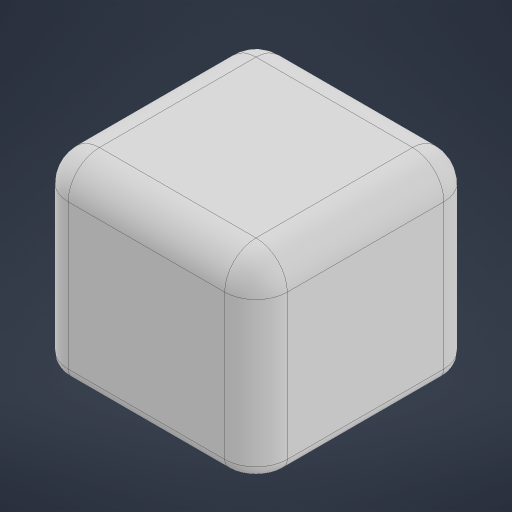
# Autodesk Inventor part: Cap
Saved by Autodesk Inventor 2024.1 (Build 281209000, 209)
## iProperties
Created: 2024-04-25
Part Number: Cap
Material: Generic
Document SubType Name: Modeling
Designer: Tim Jäger
Density: 1 g/cm^3
Appearance: Default
Author: Tim Jäger
## iProperties of the stored document Cap_3DPrint.ipt
Created: 2024-04-25
Part Number: Cap_3DPrint
Material: Generic
Document SubType Name: Modeling
Designer: Tim Jäger
Density: 1 g/cm^3
Appearance: Default
Author: Tim Jäger
Autodesk Inventor part; units mm, degrees
ref_plane "YZ Plane" through (0, 0, 0) normal (1, 0, 0) x (0, 1, 0)
ref_plane "XZ Plane" through (0, 0, 0) normal (0, 1, 0) x (-1, 0, 0)
ref_plane "XY Plane" through (0, 0, 0) normal (0, 0, 1) x (1, 0, 0)
sketch "Sketch1" plane through (0, 0, 0) normal (0, 1, 0) x (-1, 0, 0)
  line L0 (-10, 10) -> (10, 10)
  line L1 (10, 10) -> (10, -10)
  line L2 (10, -10) -> (-10, -10)
  line L3 (-10, -10) -> (-10, 10)
  line L4 (-10, 10) -> (10, -10) construction
  line L5 (10, 10) -> (-10, -10) construction
  line L6 (14, -10) -> (14, 10)
  line L7 (10, 14) -> (-10, 14)
  line L8 (-14, 10) -> (-14, -10)
  line L9 (-10, -14) -> (10, -14)
  arc A0 (10, -14) -> (14, -10) centre (10, -10) ccw
  arc A1 (-14, -10) -> (-10, -14) centre (-10, -10) ccw
  arc A2 (-10, 14) -> (-14, 10) centre (-10, 10) ccw
  arc A3 (14, 10) -> (10, 14) centre (10, 10) ccw
  point P0 (0, 0)
  point P1 (14, -14)
  point P2 (14, 14)
  point P3 (-14, 14)
  point P4 (-14, -14)
  dimension "d0" = 20
  dimension "d1" = 4
  dimension "d6" = 4
  constraints: 20 end point, 8 point on circle, 8 point on line, 8 tangent, 4 centre point, 4 parallel, 3 equal radius, 3 perpendicular, 2 midpoint, 1 horizontal, 3 other
  measures "d0" distance of L1.end L2.end
  measures "d1" distance between parallel lines of L1 L6
  measures "d6" radius of A0
extrude "Extrusion1" add sketch "Sketch1" along normal blind 20
sketch "Sketch2" plane through (0, 20, 0) normal (0, 1, 0) x (1, 0, 0)
  line L0 (-10, -14) -> (10, -14) projected
  line L1 (-14, 10) -> (-14, -10) projected
  line L2 (10, 14) -> (-10, 14) projected
  line L3 (14, -10) -> (14, 10) projected
  arc A0 (-10, 14) -> (-14, 10) centre (-10, 10) ccw projected
  arc A1 (-14, -10) -> (-10, -14) centre (-10, -10) ccw projected
  arc A2 (10, -14) -> (14, -10) centre (10, -10) ccw projected
  arc A3 (14, 10) -> (10, 14) centre (10, 10) ccw projected
  point P0 (0, 0)
  point P1 (-13, -13)
  point P2 (13, -13)
  point P3 (-13, 13)
  point P4 (13, 13)
  constraints: 4 other
extrude "Extrusion2" add sketch "Sketch2" along normal blind 4
fillet "Fillet1" radius 4 8 edges at (12.8284, 24, 12.8284) (14, 24, 0) (12.8284, 24, -12.8284) (0, 24, -14) (-12.8284, 24, -12.8284) (-14, 24, 0) (-12.8284, 24, 12.8284) (0, 24, 14)
fillet "Fillet2" radius 1.5 12 edges at (12.8284, 0, 12.8284) (14, 0, 0) (12.8284, 0, -12.8284) (0, 0, -14) (-12.8284, 0, -12.8284) (-14, 0, 0) (-12.8284, 0, 12.8284) (0, 0, 14) (0, 0, 10) (10, 0, 0) (0, 0, -10) (-10, 0, 0)
fillet "Fillet3" radius 1 8 edges at (10, 10.75, 10) (10.4393, 0.4393, 10.4393) (10, 10.75, -10) (10.4393, 0.4393, -10.4393) (-10, 10.75, -10) (-10.4393, 0.4393, -10.4393) (-10, 10.75, 10) (-10.4393, 0.4393, 10.4393)
fillet "Fillet4" radius 1 8 edges at (9.7071, 20, 9.7071) (0, 20, 10) (-9.7071, 20, 9.7071) (-10, 20, 0) (-9.7071, 20, -9.7071) (0, 20, -10) (9.7071, 20, -9.7071) (10, 20, 0)
body "Solid1"
